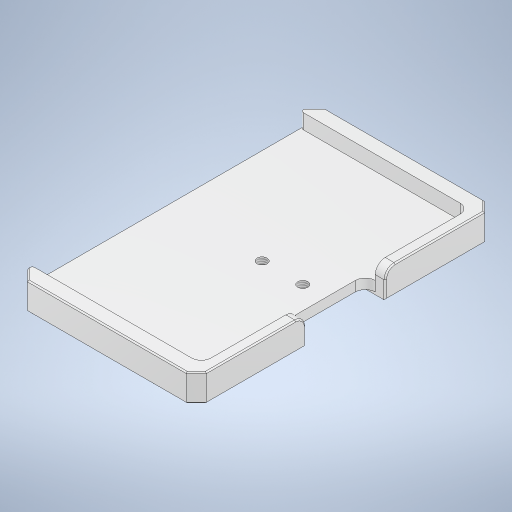
# Autodesk Inventor part: Wallet Recipe Test
Saved by Autodesk Inventor 2023.2 (Build 272271000, 271)
## iProperties
Created: 2024-03-26
Part Number: Wallet Recipe Test
Material: Aluminum 6061
Document SubType Name: Modeling
Designer: Nathan Cai
Density: 2.7 g/cm^3
Appearance: Aluminum - Flat
Author: Nathan Cai
Autodesk Inventor part; units mm, degrees
ref_plane "YZ Plane" through (0, 0, 0) normal (1, 0, 0) x (0, 1, 0)
ref_plane "XZ Plane" through (0, 0, 0) normal (0, 1, 0) x (-1, 0, 0)
ref_plane "XY Plane" through (0, 0, 0) normal (0, 0, 1) x (1, 0, 0)
sketch "Sketch1" plane through (0, 0, 0) normal (0, 1, 0) x (-1, 0, 0)
  line L0 (-28.575, 47.625) -> (28.575, 47.625)
  line L1 (28.575, 47.625) -> (28.575, -47.625)
  line L2 (28.575, -47.625) -> (-28.575, -47.625)
  line L3 (-28.575, -47.625) -> (-28.575, 47.625)
  line L4 (-28.575, 47.625) -> (28.575, -47.625) construction
  line L5 (28.575, 47.625) -> (-28.575, -47.625) construction
  point P0 (0, 0)
  dimension "d0" = 57.15
  dimension "d1" = 95.25
  constraints: 12 end point, 2 midpoint, 2 parallel, 1 horizontal, 1 perpendicular
  measures "d0" distance of L1.end L2.end
  measures "d1" distance of L0.end L1.end
extrude "Extrusion1" add sketch "Sketch1" along normal blind 8.7313
sketch "Sketch2" plane through (0, 8.7313, 0) normal (0, 1, 0) x (1, 0, 0)
  line L0 (-28.575, 47.625) -> (-28.575, -47.625) projected
  line L1 (-28.575, 0) -> (0, 0) construction
  line L2 (-28.575, -42.8625) -> (25.4, -42.8625)
  line L3 (25.4, -42.8625) -> (25.4, 42.8625)
  line L4 (25.4, 42.8625) -> (-28.575, 42.8625)
  line L5 (-28.575, 42.8625) -> (-28.575, -42.8625)
  dimension "d4" = 53.975
  dimension "d5" = 85.725
  constraints: 10 end point, 2 horizontal, 2 parallel, 1 midpoint, 1 perpendicular, 1 point on line, 1 other
  measures "d4" distance of L4.end L3.end
  measures "d5" distance of L3.end L2.end
extrude "Extrusion2" cut sketch "Sketch2" against normal blind 4.7625
fillet "Fillet1" radius 3.048 2 edges at (25.4, 6.35, 42.8625) (25.4, 6.35, -42.8625)
sketch "Sketch3" plane through (0, 0, 0) normal (0, -1, 0) x (1, 0, 0)
  line L0 (22.225, -12.7) -> (34.925, -12.7)
  line L1 (34.925, -12.7) -> (34.925, 12.7)
  line L2 (34.925, 12.7) -> (22.225, 12.7)
  line L3 (22.225, 12.7) -> (22.225, -12.7)
  line L4 (28.575, 47.625) -> (28.575, -47.625) projected
  line L5 (22.225, -12.7) -> (34.925, 12.7) construction
  line L6 (34.925, -12.7) -> (22.225, 12.7) construction
  point P0 (0, 0)
  point P1 (28.575, 0)
  dimension "d15" = 12.7
  dimension "d16" = 25.4
  constraints: 12 end point, 3 midpoint, 2 parallel, 1 horizontal, 1 perpendicular
  measures "d15" distance of L2.end L1.end
  measures "d16" distance between parallel lines of L0 L2
extrude "Extrusion3" cut sketch "Sketch3" against normal through all
sketch "Sketch4" plane through (0, 0, 0) normal (0, -1, 0) x (1, 0, 0)
  line L0 (28.575, -12.7) -> (-19.05, -12.7)
  line L1 (-19.05, -12.7) -> (-19.05, 12.7)
  line L2 (-19.05, 12.7) -> (28.575, 12.7)
  line L3 (28.575, 12.7) -> (28.575, -12.7)
  line L4 (28.575, -12.7) -> (-19.05, 12.7) construction
  line L5 (-19.05, -12.7) -> (28.575, 12.7) construction
  line L6 (0, 0) -> (22.225, 0) construction
  line L7 (22.225, 12.7) -> (22.225, -12.7) projected
  point P0 (4.7625, 0)
  point P1 (28.575, 12.7)
  point P2 (22.225, 9.525)
  point P3 (22.225, -9.525)
  dimension "d20" = 47.625
  dimension "d21" = 25.4
  constraints: 14 end point, 3 midpoint, 2 parallel, 2 point on line, 1 horizontal, 1 perpendicular
  measures "d20" distance of L1.end L2.end
  measures "d21" distance of L0.end L1.end
extrude "Extrusion4" cut sketch "Sketch4" against normal blind 0.7937
fillet "Fillet3" radius 3.175 6 edges at (22.225, 2.3813, -12.7) (26.9875, 8.7313, -12.7) (22.225, 2.3813, 12.7) (26.9875, 8.7313, 12.7) (-19.05, 0.3969, -12.7) (-19.05, 0.3969, 12.7)
sketch "Sketch5" plane through (0, 0.7937, 0) normal (0, -1, 0) x (1, 0, 0)
  line L0 (-19.05, -9.525) -> (-19.05, 9.525) projected
  line L1 (-19.05, 0) -> (22.225, 0) construction
  line L2 (22.225, 9.525) -> (22.225, -9.525) projected
  circle A0 centre (1.95, 0) radius 2
  circle A1 centre (14.95, 0) radius 2
  point P0 (0, 0)
  dimension "d25" = 4
  dimension "d26" = 21
  dimension "d29" = 13
  constraints: 2 centre point, 2 coincident, 2 end point, 2 midpoint, 1 horizontal, 1 point on line, 2 other
  measures "d25" diameter of A0
  measures "d26" distance from line of L0 A0.centre
  measures "d29" distance of A0.centre A1.centre
hole "Hole1" at (1.95, 0.7937, 0) at (14.95, 0.7937, 0) direction (0, 1, 0) diameter 3.242 end through all thread size "M4x0.7" class "6H" standard "ANSI Metric M Profile"
chamfer "Chamfer3" distance 3.175 angle 45 4 edges at (28.575, 4.3656, 47.625) (-28.575, 4.3656, 47.625) (28.575, 4.3656, -47.625) (-28.575, 4.3656, -47.625)
fillet "Fillet4" radius 0.7937 2 edges at (-28.575, 6.35, 42.8625) (-28.575, 6.35, -42.8625)
chamfer "Chamfer4" distance 0.3969 angle 45 21 edges at (28.575, 0, -28.575) (26.9875, 0, -46.0375) (0, 0, -47.625) (-26.9875, 0, -46.0375) (-28.575, 0, 0) (-26.9875, 0, 46.0375) (0, 0, 47.625) (26.9875, 0, 46.0375) (28.575, 0, 28.575) (-26.9875, 8.7312, -46.0375) (0, 8.7313, -47.625) (26.9875, 8.7312, -46.0375) (28.575, 8.7313, -30.1625) (28.575, 7.8013, -13.6299) (28.575, 2.7781, -12.7) (28.575, 8.7313, 30.1625) (28.575, 7.8013, 13.6299) (28.575, 2.7781, 12.7) (26.9875, 8.7312, 46.0375) (0, 8.7313, 47.625) (-26.9875, 8.7312, 46.0375)
body "Solid1"
